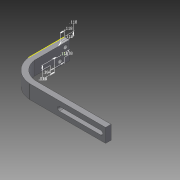
# Autodesk Inventor part: eye_cam_arm
Saved by Autodesk Inventor 2015 (Build 190159000, 159)
## iProperties
Created: 2015-06-21
Part Number: eye_cam_arm
Material: Generic
Document SubType Name: Modeling
Designer: Master
Density: 1 g/cm^3
Appearance: Default
Author: Master
Autodesk Inventor part; units mm, degrees
ref_plane "YZ Plane" through (0, 0, 0) normal (1, 0, 0) x (0, 1, 0)
ref_plane "XZ Plane" through (0, 0, 0) normal (0, 1, 0) x (-1, 0, 0)
ref_plane "XY Plane" through (0, 0, 0) normal (0, 0, 1) x (1, 0, 0)
sketch "Sketch1" plane through (0, 0, 0) normal (0, 1, 0) x (-1, 0, 0)
  line L0 (-0.4654, 17.4069) -> (54.4394, 17.4069)
  line L1 (69.5346, 3.0665) -> (69.5346, -22.5931)
  arc A0 (69.5346, 3.0665) -> (54.4394, 17.4069) centre (53.1439, 0.9282) ccw
  point P0 (0, 0)
  dimension "d0" = 70
  dimension "d1" = 40
  constraints: 4 end point, 2 point on circle, 1 centre point
  measures "d0" distance from line of L1 L0.start
  measures "d1" distance from line of L0 L1.end
sketch "Sketch2" plane through (0, 0, 0) normal (1, 0, 0) x (0, 1, 0)
  line L0 (-5, 15.4069) -> (5, 15.4069)
  line L1 (5, 15.4069) -> (5, 19.4069)
  line L2 (5, 19.4069) -> (-5, 19.4069)
  line L3 (-5, 19.4069) -> (-5, 15.4069)
  point P0 (0, 0)
  point P1 (0, 17.4069)
  dimension "d2" = 10
  dimension "d3" = 5
  dimension "d4" = 4
  dimension "d5" = 2
  constraints: 8 end point
  measures "d2" distance between parallel lines of L3 L1
  measures "d3" distance from line of point (0, 17.407) L3
  measures "d4" distance between parallel lines of L2 L0
  measures "d5" distance from line of point (0, 17.407) L2
sweep "Sweep1" add profiles "Sketch2" path "Sketch1"
sketch "Sketch3" plane through (0.4654, -5, 19.4069) normal (0, 0, 1) x (1, 0, 0)
  arc A0 (-3.5, 3.5) -> (-3.5, 6.5) centre (-3.5, 5) ccw
  arc A1 (-33.5, 6.5) -> (-33.5, 3.5) centre (-33.5, 5) ccw
  line L0 (-3.5, 3.5) -> (-33.5, 3.5)
  line L1 (-3.5, 6.5) -> (-33.5, 6.5)
  line L2 (0, 10) -> (-54.9833, 10) projected
  line L3 (0, 10) -> (0, 0) projected
  point P0 (-0.4654, 5)
  dimension "d8" = 3
  dimension "d9" = 3
  dimension "d10" = 5
  dimension "d11" = 3.5
  dimension "d12" = 30
  constraints: 4 end point, 4 point on circle, 4 vertical alignment, 2 centre point, 1 horizontal alignment
  measures "d8" diameter of A0
  measures "d9" diameter of A1
  measures "d10" distance from line of L2 A0.centre
  measures "d11" distance from line of L3 A0.centre
  measures "d12" distance of A1.centre A0.centre
extrude "Extrusion1" cut sketch "Sketch3" against normal through all
sketch "Sketch4" plane through (-71.5346, -5, -22.5931) normal (-1, 0, 0) x (0, 0, 1)
  line L0 (0, 10) -> (25.7895, 10) projected
  line L1 (0, 0) -> (0, 10) projected
  line L2 (0, 0) -> (25.7895, 0) projected
  line L3 (25.7895, 10) -> (25.7895, 0) projected
  line L4 (0, 0) -> (10, 0)
  line L5 (10, 0) -> (10, -3)
  line L6 (10, -3) -> (0, -3)
  line L7 (0, -3) -> (0, 0)
  circle A0 centre (3, 7) radius 1.5
  circle A1 centre (7, 0) radius 1.5
  point P0 (22.5931, 5)
  dimension "d15" = 3
  dimension "d16" = 10
  dimension "d17" = 3
  dimension "d18" = 3
  dimension "d19" = 3
  dimension "d20" = 3
  dimension "d21" = 3
  dimension "d22" = 3
  constraints: 8 end point, 2 centre point
  measures "d15" distance between parallel lines of L6 L2
  measures "d16" distance between parallel lines of L7 L5
  measures "d17" diameter of A0
  measures "d18" diameter of A1
  measures "d19" distance from line of L6 A1.centre
  measures "d20" distance from line of L0 A0.centre
  measures "d21" distance from line of L1 A0.centre
  measures "d22" distance from line of L5 A1.centre
extrude "Extrusion2" add sketch "Sketch4" against normal up to surface (4 mm away) contours L2 A1 L5 L6 L7 | L2 A1 picked at (6.8227, -0.4675)
extrude "Extrusion3" cut sketch "Sketch4" against normal through all contours A1 L2 | L2 A1 | A0
sketch "Sketch5" plane through (-67.5346, 5, -22.5931) normal (0, 0, -1) x (-1, 0, 0)
  line L0 (0, 0) -> (0, -13) projected
  line L1 (4, -13) -> (0, -13) projected
  line L2 (4, 0) -> (4, -13) projected
  line L3 (4, 0) -> (0, 0) projected
  circle A0 centre (5, -6.5) radius 2
  point P0 (-67.5346, -5)
  dimension "d27" = 4
  dimension "d28" = 6.5
  dimension "d31" = 1
  constraints: 1 centre point
  measures "d27" diameter of A0
  measures "d28" distance from line of A0.centre L3
  measures "d31" distance from line of L2 A0.centre
extrude "Extrusion4" cut sketch "Sketch5" against normal through all contours A0 L2 | L2 A0
equation "\"d3\" = 0.5 * d2"
equation "\"d5\" = 0.5 * d4"
body "Solid1"
